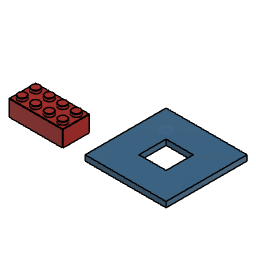
Fusion360 Models (Autodesk Fusion 360 design; units mm, degrees)
Autodesk Fusion 360 part; units mm, degrees
sketch "Sketch2" plane through (0, 0, 0) normal (0, 0, 1) x (1, 0, 0)
  line L0 (0, 0) -> (31.8, 0)
  line L1 (31.8, 0) -> (31.8, 15.8)
  line L2 (31.8, 15.8) -> (0, 15.8)
  line L3 (0, 15.8) -> (0, 0)
  dimension "d6" = 31.8
  dimension "d7" = 15.8
  constraint horizontal L0
  constraint vertical L1
  constraint horizontal L2
  constraint vertical L3
  constraint coincident L0.start L3.end
  measures "d6" distance of L0.start L0.end
  measures "d7" distance of L0.start L2.end
extrude "Extrude1" add sketch "Sketch2" along normal blind 9.6 makes body 1
sketch "Sketch3" plane through (0, 0, 9.6) normal (0, 0, 1) x (-1, 0, 0)
  line L0 (0, -15.8) -> (0, 0)
  line L1 (0, 0) -> (-31.8, 0)
  line L2 (-31.8, 0) -> (-31.8, -15.8)
  line L3 (-31.8, -15.8) -> (0, -15.8)
  circle A0 centre (-3.9, -11.9) radius 2.5
  circle A1 centre (-11.9, -11.9) radius 2.5
  circle A2 centre (-19.9, -11.9) radius 2.5
  circle A3 centre (-27.9, -11.9) radius 2.5
  circle A4 centre (-3.9, -3.9) radius 2.5
  circle A5 centre (-11.9, -3.9) radius 2.5
  circle A6 centre (-19.9, -3.9) radius 2.5
  circle A7 centre (-27.9, -3.9) radius 2.5
  dimension "d10" = 5
  dimension "d11" = 3.9
  dimension "d12" = 3.9
  dimension "d15" = -24
  dimension "d16" = 8
  measures "d10" diameter of A0
  measures "d11" distance of L3 A0.centre
  measures "d12" distance of L0 A0.centre
extrude "Extrude2" add sketch "Sketch3" along normal blind 1.7 contours A0 | A1 | A2 | A3 | A4 | A5 | A6 | A7 bodies 1
shell "Shell1" thickness 1.49 removed faces 1 at (21.2, 5.2667, 0) on bodies 1
sketch "Sketch4" plane through (0, 0, 8.11) normal (0, 0, -1) x (1, 0, 0)
  circle A0 centre (3.9, -3.9) radius 1.01
  circle A1 centre (27.9, -3.9) radius 1.01
  circle A2 centre (11.9, -11.9) radius 1.01
  circle A3 centre (19.9, -3.9) radius 1.01
  circle A4 centre (3.9, -11.9) radius 1.01
  circle A5 centre (27.9, -11.9) radius 1.01
  circle A6 centre (19.9, -11.9) radius 1.01
  circle A7 centre (11.9, -3.9) radius 1.01
  line L0 (1.49, -1.49) -> (1.49, -14.31)
  line L1 (1.49, -14.31) -> (30.31, -14.31)
  line L2 (30.31, -14.31) -> (30.31, -1.49)
  line L3 (30.31, -1.49) -> (1.49, -1.49)
  circle A8 centre (3.9, -3.9) radius 2.5
  circle A9 centre (11.9, -11.9) radius 2.5
  circle A10 centre (3.9, -11.9) radius 2.5
  circle A11 centre (11.9, -3.9) radius 2.5
  circle A12 centre (7.9, -7.9) radius 3.1569
  circle A13 centre (7.9, -7.9) radius 2.1569
  circle A14 centre (15.9, -7.9) radius 2.1569
  circle A15 centre (15.9, -7.9) radius 3.1569
  circle A16 centre (23.9, -7.9) radius 2.1569
  circle A17 centre (23.9, -7.9) radius 3.1569
  line L4 (11.9, -3.9) -> (11.1858, -4.6142)
  line L5 (5.6678, -10.1322) -> (3.9, -11.9)
  dimension "d20" = 5
  dimension "d21" = 5
  dimension "d22" = 5
  dimension "d23" = 5
  dimension "d24" = -1
  dimension "d27" = 16
  dimension "d28" = 0
  constraint concentric A0 A8
  constraint concentric A2 A9
  constraint concentric A4 A10
  constraint concentric A7 A11
  constraint coincident A7.centre A11.centre
  constraint coincident A4.centre A10.centre
  constraint tangent A8 A12
  constraint collinear L4 L5
  constraint coincident A12.centre L4
  constraint coincident A7 L4.end
  constraint coincident A10 L5.start
  measures "d20" diameter of A8
  measures "d21" diameter of A9
  measures "d22" diameter of A10
  measures "d23" diameter of A11
extrude "Extrude3" add sketch "Sketch4" along normal blind 8.1 contours A12 | A15 | A17 bodies 1
fillet "Fillet1" radius 0.2 22 edges at (15.9, 15.8, 9.6) (15.9, 0, 9.6) (0, 7.9, 9.6) (30.2308, 4.804, 11.3) (30.2308, 12.804, 11.3) (22.2308, 4.804, 11.3) (22.2308, 12.804, 11.3) (14.2308, 12.804, 11.3) (14.2308, 4.804, 11.3) (6.2308, 12.804, 11.3) (6.2308, 4.804, 11.3) (0, 0, 4.8) (31.8, 0, 4.8) (31.8, 15.8, 4.8) (31.8, 7.9, 9.6) (0, 15.8, 4.8) (12.9568, 9.0416, 0.01) (13.8891, 7.12, 0.01) (20.9568, 9.0416, 0.01) (21.8891, 7.12, 0.01) (4.9568, 9.0416, 0.01) (5.8891, 7.12, 0.01) on bodies 1
sketch "Sketch5" plane through (0, 0, 0) normal (0, 0, 1) x (1, 0, 0)
  line L0 (45, 0) -> (92.8, 0)
  line L1 (92.8, 0) -> (92.8, 47.8)
  line L2 (92.8, 47.8) -> (45, 47.8)
  line L3 (45, 47.8) -> (45, 0)
  line L4 (60.9, 15.9) -> (76.9, 15.9)
  line L5 (76.9, 15.9) -> (76.9, 31.9)
  line L6 (76.9, 31.9) -> (60.9, 31.9)
  line L7 (60.9, 31.9) -> (60.9, 15.9)
  dimension "d32" = 47.8
  dimension "d33" = 47.8
  dimension "d34" = 16
  dimension "d35" = 16
  dimension "d36" = 15.9
  dimension "d37" = 15.9
  constraint horizontal L0
  constraint vertical L1
  constraint horizontal L2
  constraint vertical L3
  constraint horizontal L4
  constraint vertical L5
  constraint horizontal L6
  constraint vertical L7
  measures "d32" distance of L0.start L0.end
  measures "d33" distance of L0.start L2.end
  measures "d34" distance of L4.start L4.end
  measures "d35" distance of L4.start L6.end
  measures "d36" distance of L0 L4
  measures "d37" distance of L3 L7
extrude "Extrude4" add sketch "Sketch5" along normal blind 3.2 separate body makes body 2
shell "Shell2" thickness 1.2 removed faces 1 at (87.5, 26.5667, 0) on bodies 2
sketch "Sketch6" plane through (0, 0, 2) normal (0, 0, -1) x (1, 0, 0)
  line L0 (59.7, -33.1) -> (59.7, -14.7)
  line L1 (59.7, -14.7) -> (78.1, -14.7)
  line L2 (78.1, -14.7) -> (78.1, -33.1)
  line L3 (78.1, -33.1) -> (59.7, -33.1)
  line L4 (46.2, -1.2) -> (46.2, -46.6)
  line L5 (46.2, -46.6) -> (91.6, -46.6)
  line L6 (91.6, -46.6) -> (91.6, -1.2)
  line L7 (91.6, -1.2) -> (46.2, -1.2)
  circle A0 centre (53, -8) radius 2.4
  circle A1 centre (53, -8) radius 3.255
  circle A2 centre (61, -8) radius 2.4
  circle A3 centre (61, -8) radius 3.255
  circle A4 centre (69, -8) radius 2.4
  circle A5 centre (69, -8) radius 3.255
  circle A6 centre (77, -8) radius 2.4
  circle A7 centre (77, -8) radius 3.255
  circle A8 centre (85, -8) radius 2.4
  circle A9 centre (85, -8) radius 3.255
  circle A10 centre (53, -16) radius 2.4
  circle A11 centre (53, -16) radius 3.255
  circle A12 centre (85, -16) radius 2.4
  circle A13 centre (85, -16) radius 3.255
  circle A14 centre (53, -24) radius 2.4
  circle A15 centre (53, -24) radius 3.255
  circle A16 centre (85, -24) radius 2.4
  circle A17 centre (85, -24) radius 3.255
  circle A18 centre (53, -32) radius 2.4
  circle A19 centre (53, -32) radius 3.255
  circle A20 centre (85, -32) radius 2.4
  circle A21 centre (85, -32) radius 3.255
  circle A22 centre (53, -40) radius 2.4
  circle A23 centre (53, -40) radius 3.255
  circle A24 centre (61, -40) radius 2.4
  circle A25 centre (61, -40) radius 3.255
  circle A26 centre (69, -40) radius 2.4
  circle A27 centre (69, -40) radius 3.255
  circle A28 centre (77, -40) radius 2.4
  circle A29 centre (77, -40) radius 3.255
  circle A30 centre (85, -40) radius 2.4
  circle A31 centre (85, -40) radius 3.255
  dimension "d41" = 4.8
  dimension "d42" = 6.51
  dimension "d45" = 32
  dimension "d46" = -32
  constraint concentric A0 A1
  measures "d41" diameter of A0
  measures "d42" diameter of A1
extrude "Extrude5" add sketch "Sketch6" along normal blind 2 contours A1 | A3 | A5 | A7 | A9 | A11 | A13 | A15 | A17 | A19 | A21 | A23 | A25 | A27 | A29 | A31 bodies 2
fillet "Fillet2" radius 0.2 32 edges at (65.9653, 41.1771, 0) (73.9653, 41.1771, 0) (66.7624, 39.1321, 0) (74.7624, 39.1321, 0) (57.9653, 41.1771, 0) (58.7624, 39.1321, 0) (50.7624, 39.1321, 0) (49.9653, 41.1771, 0) (49.9653, 33.1771, 0) (50.7624, 31.1321, 0) (50.7624, 23.1321, 0) (49.9653, 25.1771, 0) (49.9653, 17.1771, 0) (50.7624, 15.1321, 0) (49.9653, 9.1771, 0) (50.7624, 7.1321, 0) (58.7624, 7.1321, 0) (57.9653, 9.1771, 0) (65.9653, 9.1771, 0) (66.7624, 7.1321, 0) (73.9653, 9.1771, 0) (74.7624, 7.1321, 0) (81.9653, 9.1771, 0) (82.7624, 7.1321, 0) (81.9653, 17.1771, 0) (82.7624, 15.1321, 0) (82.7624, 23.1321, 0) (81.9653, 25.1771, 0) (81.9653, 33.1771, 0) (82.7624, 31.1321, 0) (81.9653, 41.1771, 0) (82.7624, 39.1321, 0) on bodies 2
sketch "Sketch7" plane through (0, 0, 0) normal (0, 0, -1) x (1, 0, 0)
  circle A0 centre (53, -40) radius 2.6
  circle A1 centre (53, -40) radius 3.055
equation "d45 = ( 8 * 4 ) * 1 mm"
equation "d46 = ( -8 * 4 ) * 1 mm"
